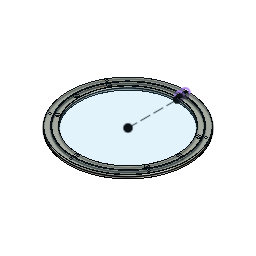
300mm Lazy Susan (Autodesk Fusion 360 design; units mm, degrees)
Autodesk Fusion 360 part; units mm, degrees
sketch "Rings" plane through (0, 0, 0) normal (0, 0, 1) x (1, 0, 0) in component "Lazy Susan"
  circle A0 centre (0, 0) radius 150
  circle A1 centre (0, 0) radius 137
  circle A2 centre (0, 0) radius 136
  circle A3 centre (0, 0) radius 123
  line L0 (0, 0) -> (0, 150) construction
  point P0 (0, 143.5)
  point P1 (0, 129.5)
  point P2 (0, 123)
  dimension "d6" = 300
  dimension "d7" = 13
  dimension "d8" = 13
  dimension "d9" = 1
  dimension "d17" = 6.5
  dimension "d18" = 6.5
  constraint coincident A0.centre A1.centre
  constraint concentric A0 A2
  constraint concentric A1 A3
  constraint coincident A0 L0.end
  constraint vertical L0
  constraint coincident L0 P0
  constraint coincident L0 P1
  constraint coincident A3 P2
  constraint coincident L0 P2
  measures "d6" diameter of A0
  measures "d7" distance of A0 A1
  measures "d8" distance of A2 A3
  measures "d9" distance of A1 A2
  measures "d17" distance of L0.end P0
  measures "d18" distance of P1 P2
extrude "Extrude1" add sketch "Rings" along normal mid plane 10.2 contours A0 makes body 1 in component "Outer Ring"
extrude "Extrude1'" add sketch "Rings" along normal mid plane 10.2 separate body contours A2 makes body 2 in component "Inner Ring"
chamfer "Chamfer1" distance 0.5 angle 45 4 edges at (-126.7965, -49.1797, 5.1) (-114.6763, 44.4787, 5.1) (-126.7965, 49.1797, -5.1) (-114.6763, -44.4787, -5.1) on bodies 2 in component "Inner Ring"
chamfer "Chamfer1'" distance 0.5 angle 45 4 edges at (-139.8491, -54.2423, 5.1) (-127.7288, 49.5413, 5.1) (-139.8491, 54.2423, -5.1) (-127.7288, -49.5413, -5.1) on bodies 1 in component "Outer Ring"
sketch "Holes" plane through (0, 0, 5.1) normal (0, 0, 1) x (-1, 0, 0) in component "Lazy Susan"
  circle A0 centre (0, 0) radius 149.5
  circle A1 centre (0, 0) radius 137.5
  point P0 (0, -143.5)
  point P1 (0, -129.5)
hole "Hole1" at (0, 143.5, 5.1) direction (0, 0, -1) diameter 5.1054 end through all bodies 1 in component "Outer Ring"
hole "Hole1'" at (0, 129.5, 5.1) direction (0, 0, -1) diameter 5.1054 depth 10.2108 tip angle 180 countersink diameter 9.779 countersink angle 82 bodies 2 in component "Inner Ring"
pattern_circular "C-Pattern1" count 6 over 360 about axis through (0, 0, 1.75) along (0, 0, 1) of "Hole1" in component "Outer Ring"
pattern_circular "C-Pattern1'" count 4 over 360 about axis through (0, 0, 1.75) along (0, 0, 1) of "Hole1'" in component "Inner Ring"
pattern_circular "C-Pattern2" count 6 over 360 about axis through (0, 0, 1.75) along (0, 0, 1) of "Hole1'" in component "Inner Ring"
component "Lazy Susan" placed x (1, 0, 0) y (0, 1, 0) z (0, 0, 1) at (0, 0, 0)
component "Outer Ring" placed x (1, 0, 0) y (0, 1, 0) z (0, 0, 1) at (0, 0, 0) in component "Lazy Susan"
component "Inner Ring" placed x (1, 0, 0) y (0, 1, 0) z (0, 0, 1) at (0, 0, 0) in component "Lazy Susan"
equation "LAZY_SUSAN_OD = 300 mm" comment "OD of the \"12-inch\" Lazy Susan"
equation "LAZY_SUSAN_OUTER_RING = 13 mm" comment "Width of outer ring"
equation "LAZY_SUSAN_INNER_RING = 13 mm" comment "Width of the inner ring"
equation "LAZY_SUSAN_GAP = 1 mm" comment "Gap between rings"
equation "LAZY_SUSAN_THICKNESS = 10.2 mm" comment "Thickness of the rings"
equation "d6 = LAZY_SUSAN_OD"
equation "d7 = LAZY_SUSAN_OUTER_RING"
equation "d8 = LAZY_SUSAN_INNER_RING"
equation "d9 = LAZY_SUSAN_GAP"
equation "d10 = LAZY_SUSAN_THICKNESS"
equation "d12 = LAZY_SUSAN_THICKNESS"
equation "CHAMFER = 0.5 mm" comment "Edge chamfer on rings"
equation "d15 = CHAMFER"
equation "d16 = CHAMFER"
equation "d17 = LAZY_SUSAN_OUTER_RING / 2"
equation "d18 = LAZY_SUSAN_INNER_RING / 2"
